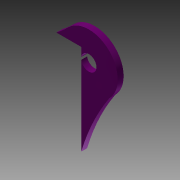
# Autodesk Inventor part: rumahbearing
Saved by Autodesk Inventor 2015 (Build 190159000, 159)
## iProperties
Created: 2015-01-18
Part Number: rumahbearing
Material: Generic
Document SubType Name: Modeling
Designer: Rafi Kurnia Putra
Density: 1 g/cm^3
Appearance: Smooth - Purple
Author: Rafi Kurnia Putra
Autodesk Inventor part; units mm, degrees
ref_plane "YZ Plane" through (0, 0, 0) normal (1, 0, 0) x (0, 1, 0)
ref_plane "XZ Plane" through (0, 0, 0) normal (0, 1, 0) x (-1, 0, 0)
ref_plane "XY Plane" through (0, 0, 0) normal (0, 0, 1) x (1, 0, 0)
sketch "Sketch1" plane through (0, 0, 0) normal (0, 1, 0) x (-1, 0, 0)
  arc A0 (-43.442, 61.4074) -> (-43.442, 60.3658) centre (-46.65, 60.8866) ccw
  arc A1 (-43.9419, 28.3111) -> (-55.3297, 52.2069) centre (-134.1138, 0) ccw
  arc A2 (-37.9127, 69.5084) -> (-55.3297, 52.2069) centre (-46.65, 60.8866) ccw
  arc A3 (-37.9703, 69.5664) -> (-33.5565, 65.6366) centre (-4.3624, 102.8704) ccw
  arc A4 (-43.442, 26.6668) -> (-55.3297, 52.2069) centre (-134.1138, 0) ccw
  arc A5 (-43.9419, 28.3111) -> (-55.3297, 52.2069) centre (-134.1138, 0) ccw
  arc A6 (-37.9703, 69.5664) -> (-55.3297, 52.2069) centre (-46.65, 60.8866) ccw
  arc A7 (-37.9703, 69.5664) -> (-32.9073, 65.1366) centre (-4.3624, 102.8704) ccw
  arc A8 (-43.442, 61.4075) -> (-43.442, 60.3658) centre (-46.65, 60.8866) ccw
  arc A9 (-43.442, 61.4074) -> (-43.442, 60.3658) centre (-46.65, 60.8866) ccw
  line L0 (-43.442, 26.6668) -> (-43.442, 60.8866)
  line L1 (-43.442, 60.8866) -> (-43.442, 65.1366)
  line L2 (-43.442, 65.1366) -> (-32.9073, 65.1366)
  line L3 (-43.442, 65.1366) -> (-43.442, 26.6668)
  arc A10 (-43.442, 26.6668) -> (-55.3297, 52.2069) centre (-134.1139, -0.0001) ccw
  arc A11 (-37.9703, 69.5664) -> (-55.3297, 52.2069) centre (-46.65, 60.8866) ccw
  arc A12 (-37.9703, 69.5664) -> (-32.9073, 65.1366) centre (-4.3624, 102.8704) ccw
  line L4 (-32.9073, 65.1366) -> (-43.442, 65.1366)
  arc A13 (-43.442, 61.4074) -> (-43.442, 60.3658) centre (-46.65, 60.8866) ccw
  point P0 (0, 0)
  point P1 (-43.9419, 28.3111)
  constraints: 34 point on circle, 14 centre point, 10 end point, 8 point on line, 3 coincident, 2 tangent, 1 collinear, 1 horizontal, 1 vertical
extrude "Extrusion2" add sketch "Sketch1" along normal blind 2.5 contours A0 L0 A4 A1 A2 A3 A7 L2 L1
body "Solid2"
